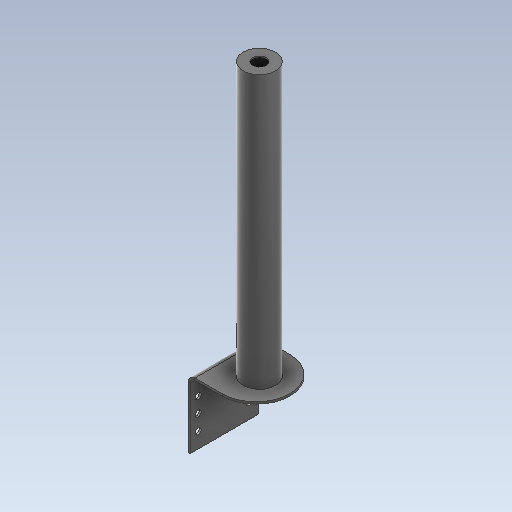
# Autodesk Inventor part: Pole
Saved by Autodesk Inventor 2020 (Build 240168000, 168)
## iProperties
Created: 2021-07-08
Part Number: Pole
Material: Steel, Carbon
Document SubType Name: Sheet Metal
Designer: Simon.Alvarez
Density: 7.85 g/cm^3
Sheet Metal Rule: Default_mm
Appearance: Semi-Polished
Width: 100.000 mm
Bolt_Width: 75.000 mm
Bolt_Height: 45.000 mm
Clamp_Bolt_Space: 35.000 mm
Tube_Dia: 48.000 mm
Author: Simon.Alvarez
Autodesk Inventor part; units mm, degrees
ref_plane "YZ Plane" through (0, 0, 0) normal (1, 0, 0) x (0, 1, 0)
ref_plane "XZ Plane" through (0, 0, 0) normal (0, 1, 0) x (-1, 0, 0)
ref_plane "XY Plane" through (0, 0, 0) normal (0, 0, 1) x (1, 0, 0)
sketch "Sketch1" plane through (0, 0, 0) normal (0, 1, 0) x (-1, 0, 0)
  line L0 (-45, 50) -> (45, 50)
  line L1 (45, 50) -> (45, -50)
  line L2 (45, -50) -> (-45, -50)
  line L3 (-45, -50) -> (-45, 50)
  line L4 (-45, 50) -> (45, -50) construction
  line L5 (45, 50) -> (-45, -50) construction
  point P0 (0, 0)
  dimension "d0" = 90
  dimension "d1" = 100
  constraints: 12 end point, 2 midpoint, 2 parallel, 1 horizontal, 1 perpendicular
  measures "d0" distance of L1.end L2.end
  measures "d1" distance of L0.end L1.end
extrude "Extrusion1" add sketch "Sketch1" along normal blind 3
sketch "Sketch2" plane through (-52, -7, -50) normal (-1, 0, 0) x (0, -1, 0)
  line L0 (0, 100) -> (0, 0)
  line L1 (0, 0) -> (90, 0)
  line L2 (90, 0) -> (90, 100)
  line L3 (90, 100) -> (0, 100)
  constraints: 6 end point, 1 horizontal, 1 perpendicular, 1 vertical
edge flange "Flange1" height 100 angle 90 thickness 3 bend radius 7 thickness toward (-1, 0, 0) relief tear relief width 3 relief depth 1.5 edges at (-45, 0, 0) wall of the first edge with corners at (-52, -7, 50) (-52, -7, -50) (-52, -97, -50) (-52, -97, 50)
bend "Bend1"
corner "Corner1"
fillet "Fillet1" radius 50 2 edges at (45, 1.5, 50) (45, 1.5, -50)
sketch "Sketch3" plane through (0, 3, 0) normal (0, 1, 0) x (1, 0, 0)
  circle A0 centre (0, 0) radius 24
  circle A1 centre (0, 0) radius 22.35
  dimension "d16" = 48
  dimension "d17" = 1.65
  constraints: 2 centre point, 1 coincident
  measures "d16" diameter of A0
  measures "d17" radial gap between concentric circles of A0 A1
extrude "Extrusion2" add sketch "Sketch3" along normal blind 400
sketch "Sketch4" plane through (0, 403, 0) normal (0, 1, 0) x (1, 0, 0)
  circle A0 centre (0, 0) radius 24
  constraints: 1 centre point, 1 coincident
extrude "Extrusion3" add sketch "Sketch4" along normal blind 1.65
sketch "Sketch5" plane through (-55, -97, -50) normal (-1, 0, 0) x (0, 0, 1)
  line L0 (13.0795, 22.5) -> (88.0795, 22.5)
  line L1 (88.0795, 22.5) -> (88.0795, 67.5)
  line L2 (88.0795, 67.5) -> (13.0795, 67.5)
  line L3 (13.0795, 67.5) -> (13.0795, 22.5)
  line L4 (13.0795, 22.5) -> (88.0795, 67.5) construction
  line L5 (88.0795, 22.5) -> (13.0795, 67.5) construction
  line L6 (100, 90) -> (100, 0) projected
  point P0 (50, 97)
  point P1 (50.5795, 45)
  point P2 (50.5795, 45)
  point P3 (100, 45)
  point P4 (13.0795, 45)
  point P5 (88.0795, 45)
  dimension "d22" = 75
  dimension "d23" = 45
  constraints: 12 end point, 6 midpoint, 4 coincident, 2 parallel, 1 horizontal, 1 horizontal alignment, 1 perpendicular
  measures "d22" distance of L1.end L2.end
  measures "d23" distance of L0.end L1.end
hole "Hole1" at (-55, -29.5, -36.9205) at (-55, -52, -36.9205) at (-55, -74.5, -36.9205) at (-55, -29.5, 38.0795) at (-55, -52, 38.0795) at (-55, -74.5, 38.0795) direction (1, 0, 0) diameter 9 depth 3 tip angle 118 clearance for "Hex Head Cap Screw" size "M8" standard "Ansi Metric M Profile"
sketch "Sketch6" plane through (0, 0, 0) normal (1, 0, 0) x (0, 1, 0)
  line L0 (38, -15) -> (68, -15)
  line L1 (83, 0) -> (83, 0)
  line L2 (68, 15) -> (38, 15)
  line L3 (23, 0) -> (23, 0)
  line L4 (23, -15) -> (83, 15) construction
  line L5 (83, -15) -> (23, 15) construction
  line L6 (3, -50) -> (3, 50) projected
  arc A0 (68, -15) -> (83, 0) centre (68, 0) ccw
  arc A1 (83, 0) -> (68, 15) centre (68, 0) ccw
  arc A2 (38, 15) -> (23, 0) centre (38, 0) ccw
  arc A3 (23, 0) -> (38, -15) centre (38, 0) ccw
  point P0 (0, 0)
  point P1 (53, 0)
  point P2 (53, 0)
  point P3 (3, 0)
  point P4 (83, 0)
  point P5 (23, 0)
  dimension "d31" = 20
  dimension "d32" = 60
  dimension "d33" = 30
  dimension "d34" = 15
  constraints: 12 end point, 8 point on circle, 8 point on line, 8 tangent, 4 centre point, 4 midpoint, 2 concentric, 2 parallel, 1 equal radius, 1 horizontal, 1 horizontal alignment, 1 perpendicular
  measures "d31" distance between parallel lines of L6 L3
  measures "d32" distance of L4.end L5.end
  measures "d33" distance of L5.start L4.end
  measures "d34" radius of A0
extrude "Extrusion4" cut sketch "Sketch6" against normal through all
sketch "Sketch7" plane through (0, 404.65, 0) normal (0, 1, 0) x (1, 0, 0)
  point P0 (0, 0)
  point P1 (0, 0)
  constraints: 1 coincident
hole "Hole2" at (0, 404.65, 0) direction (0, -1, 0) diameter 20 depth 10 tip angle 118
sketch "Sketch8" plane through (0, 0, 0) normal (1, 0, 0) x (0, 1, 0)
  line L0 (404.65, -24) -> (404.65, 24) projected
  point P0 (0, 0)
  point P1 (384.65, 0)
  dimension "d44" = 20
  measures "d44" distance from line of point (384.65, 0) L0
hole "Hole3" at (0, 384.65, 0) direction (-1, 0, 0) diameter 4.917 end through all thread size "M6x1" class "6H" standard "ANSI Metric M Profile"
pattern_linear "Rectangular Pattern1" count 9 spacing 35 along (0, -1, 0) of "Hole3"
equation "\"d16\" = Tube_Dia"
equation "\"d29\" = Thickness"
equation "\"d4\" = Thickness"
equation "\"d5\" = BendReliefWidth"
equation "\"d6\" = BendReliefDepth"
equation "\"d7\" = MinimumRemnant"
equation "\"d8\" = TransitionRadius"
equation "\"d12\" = CornerReliefSize"
equation "\"d13\" = GapSize"
equation "\"d14\" = JacobiRadiusSize"
equation "\"BendRadius\" = Thickness"
equation "\"BendReliefWidth\" = Thickness"
equation "\"BendReliefDepth\" = 0.5 * Thickness"
equation "\"CornerReliefSize\" = 4 * Thickness"
equation "\"MinimumRemnant\" = 2 * Thickness"
equation "\"TransitionRadius\" = BendRadius"
equation "\"JacobiRadiusSize\" = BendRadius"
equation "\"GapSize\" = Thickness"
equation "\"Width\" = 100"
equation "\"Bolt_Width\" = 75"
equation "\"Bolt_Height\" = 45"
equation "\"Clamp_Bolt_Space\" = 35"
equation "\"Tube_Dia\" = 48"
equation "\"Thickness\" = 3"
body "Solid1"
